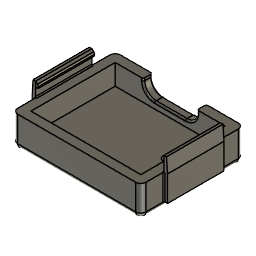
ด้านบน (Autodesk Fusion 360 design; units mm, degrees)
Autodesk Fusion 360 part; units mm, degrees
note: some values were not read from the file. Set by a fixed rule: which sketch regions a step uses.
sketch "Sketch1" plane through (0, 0, 0) normal (0, 0, 1) x (1, 0, 0)
  line L0 (0, 0) -> (21.4, 0)
  line L1 (21.4, 0) -> (21.4, 16.4)
  line L2 (21.4, 16.4) -> (0, 16.4)
  line L3 (0, 16.4) -> (0, 0)
  line L4 (-1.8, -1.8) -> (23.2, -1.8)
  line L5 (23.2, -1.8) -> (23.2, 18.2)
  line L6 (23.2, 18.2) -> (-1.8, 18.2)
  line L7 (-1.8, 18.2) -> (-1.8, -1.8)
  dimension "d1" = 21.4
  dimension "d2" = 16.4
  dimension "d3" = 25
  dimension "d4" = 20
  dimension "d5" = 1.8
  dimension "d6" = 1.8
  constraint horizontal L0
  constraint vertical L1
  constraint horizontal L2
  constraint vertical L3
  constraint coincident L0.start L3.end
  constraint horizontal L4
  constraint vertical L5
  constraint horizontal L6
  constraint vertical L7
  measures "d1" distance of L0.start L0.end
  measures "d2" distance of L0.start L2.end
  measures "d3" distance of L4.start L4.end
  measures "d4" distance of L4.start L6.end
  measures "d5" distance of L3 L7
  measures "d6" distance of L2 L6
extrude "Extrude1" add sketch "Sketch1" along normal blind 6 makes body 1
extrude "Extrude2" add sketch "Sketch1" along normal blind 2 contours L0 L1 L2 L3 bodies 1
fillet "Fillet1" radius 1 7 edges at (23.2, 8.2, 0) (10.7, 18.2, 0) (23.2, 18.2, 3) (23.2, -1.8, 3) (10.7, -1.8, 0) (-1.8, 8.2, 0) (-1.8, -1.8, 3) on bodies 1
fillet "Fillet2" radius 1 2 edges at (-1.5071, 17.9071, 0.2929) (-1.8, 18.2, 3.5) on bodies 1
sketch "Sketch3" plane through (23.2, 0, 0) normal (1, 0, 0) x (0, 1, 0)
  line L0 (-0.8, 6) -> (-0.8, 1)
  line L1 (-0.8, 1) -> (17.2, 1)
  line L2 (17.2, 1) -> (17.2, 6)
  line L3 (17.2, 6) -> (-0.8, 6)
  line L4 (2.7, 6) -> (13.7, 6)
  line L5 (13.7, 6) -> (13.7, 1)
  line L6 (13.7, 1) -> (2.7, 1)
  line L7 (2.7, 1) -> (2.7, 6)
  line L8 (2.7, 6) -> (13.7, 1) construction
  line L9 (13.7, 6) -> (2.7, 1) construction
  point P0 (8.2, 3.5)
  dimension "d15" = 11
  dimension "d16" = 5
  constraint horizontal L4
  constraint perpendicular L4 L5
  constraint parallel L4 L6
  constraint parallel L5 L7
  constraint coincident L8 P0
  constraint coincident L9 P0
  measures "d15" distance of L5.end L6.end
  measures "d16" distance of L4.end L5.end
extrude "Extrude3" add sketch "Sketch3" along normal blind 1 separate body contours L1 L3 L4 L5 L6 L7 makes body 2
sketch "Sketch4" plane through (-1.8, 0, 0) normal (-1, 0, 0) x (0, -1, 0)
  line L0 (-17.2, 6) -> (-17.2, 1)
  line L1 (-17.2, 1) -> (0.8, 1)
  line L2 (0.8, 1) -> (0.8, 6)
  line L3 (0.8, 6) -> (-17.2, 6)
  line L4 (-13.7, 6) -> (-2.7, 6)
  line L5 (-2.7, 6) -> (-2.7, 1)
  line L6 (-2.7, 1) -> (-13.7, 1)
  line L7 (-13.7, 1) -> (-13.7, 6)
  line L8 (-13.7, 6) -> (-2.7, 1) construction
  line L9 (-2.7, 6) -> (-13.7, 1) construction
  point P0 (-8.2, 3.5)
  dimension "d19" = 11
  dimension "d20" = 5
  constraint horizontal L4
  constraint perpendicular L4 L5
  constraint parallel L4 L6
  constraint parallel L5 L7
  constraint coincident L8 P0
  constraint coincident L9 P0
  measures "d19" distance of L5.end L6.end
  measures "d20" distance of L4.end L5.end
extrude "Extrude4" add sketch "Sketch4" along normal blind 1 separate body contours L1 L3 L4 L5 L6 L7 makes body 3
extrude "Extrude5" add 2 faces at (-2.4667, 6.3667, 6) (23.8667, 10.0333, 6) along direction (0, 0, 1) blind 2.8 on bodies 2 3 bodies 1 3 2
sketch "Sketch5" plane through (0, 2.7, 0) normal (0, -1, 0) x (1, 0, 0)
  line L0 (-1.8, 1) -> (-1.8, 6)
  line L1 (-1.8, 6) -> (-1.8, 8.8)
  line L2 (-1.8, 8.8) -> (-2.8, 8.8)
  line L3 (-2.8, 8.8) -> (-2.8, 1)
  line L4 (-2.8, 1) -> (-1.8, 1)
  line L5 (-1.8, 8.8) -> (-1.3, 8.8)
  line L6 (-1.3, 8.8) -> (-1.3, 7.8)
  line L7 (-1.3, 7.8) -> (-1.8, 7.8)
  line L8 (-1.8, 7.8) -> (-1.8, 8.8)
  dimension "d25" = 0.5
  dimension "d26" = 1
  constraint horizontal L5
  constraint vertical L6
  constraint horizontal L7
  constraint vertical L8
  constraint coincident L1.end L2.start
  measures "d25" distance of L1.end L5.end
  measures "d26" distance of L1.end L7.end
sketch "Sketch6" plane through (0, 2.7, 0) normal (0, -1, 0) x (1, 0, 0)
  line L0 (23.2, 6) -> (23.2, 1)
  line L1 (23.2, 1) -> (24.2, 1)
  line L2 (24.2, 1) -> (24.2, 8.8)
  line L3 (24.2, 8.8) -> (23.2, 8.8)
  line L4 (23.2, 8.8) -> (23.2, 6)
  line L5 (23.2, 8.8) -> (22.7, 8.8)
  line L6 (22.7, 8.8) -> (22.7, 7.8)
  line L7 (22.7, 7.8) -> (23.2, 7.8)
  line L8 (23.2, 7.8) -> (23.2, 8.8)
  dimension "d27" = 0.5
  dimension "d28" = 1
  constraint horizontal L5
  constraint vertical L6
  constraint horizontal L7
  constraint vertical L8
  constraint coincident L3.end L4.start
  measures "d27" distance of L3.end L5.end
  measures "d28" distance of L3.end L7.end
extrude "Extrude6" add sketch "Sketch6" sketch "Sketch5" against normal blind 11 separate body contours L4 L5 L6 L7 L8 of sketch 2 contours L1 L5 L6 L7 L8 makes body 4 at (22.7, 6.3667, 8.4667) makes body 5 at (-1.3, 6.3667, 8.4667)
sketch "Sketch7" plane through (0, 2.7, 0) normal (0, -1, 0) x (1, 0, 0)
  line L0 (-1.8, 1) -> (-1.8, 6)
  line L1 (-1.8, 6) -> (-1.8, 8.8)
  line L2 (-1.8, 8.8) -> (-2.8, 8.8)
  line L3 (-2.8, 8.8) -> (-2.8, 1)
  line L4 (-2.8, 1) -> (-1.8, 1)
  line L5 (-1.8, 6) -> (-2.4875, 6)
  line L6 (-2.4875, 6) -> (-2.8, 6)
  line L7 (-2.4875, 5.8364) -> (-2.4875, 1)
  line L8 (-2.4875, 6) -> (-2.3, 8.8)
  line L9 (-2.4875, 5.8364) -> (-2.4875, 6)
  constraint midpoint L2 L8.end
  constraint coincident L0.end L1.start
  constraint perpendicular L0 L5
  constraint coincident L3 L6.end
  constraint perpendicular L3 L6
  constraint coincident L4 L7.end
  constraint perpendicular L4 L7
  constraint perpendicular L5 L9
chamfer "Chamfer1" distance 0.5 angle 45 1 edges at (22.7, 8.2, 8.8) on bodies 4
chamfer "Chamfer2" distance 0.5 angle 45 1 edges at (-1.3, 8.2, 8.8) on bodies 5
fillet "Fillet6" radius 0.5 1 edges at (22.7, 8.2, 8.3) on bodies 4 5
fillet "Fillet6" radius 0.5 1 edges at (-1.3, 8.2, 8.3) on bodies 4 5
extrude "Extrude7" cut sketch "Sketch7" against normal blind 18.339 contours L2 L3 L6 L8 bodies 1
sketch "Sketch8" plane through (0, 2.7, 0) normal (0, -1, 0) x (1, 0, 0)
  line L0 (23.2, 6) -> (23.2, 1)
  line L1 (23.2, 1) -> (24.2, 1)
  line L2 (24.2, 1) -> (24.2, 8.8)
  line L3 (24.2, 8.8) -> (23.2, 8.8)
  line L4 (23.2, 8.8) -> (23.2, 6)
  line L5 (23.8875, 6) -> (23.7, 8.8)
  line L6 (23.2, 6) -> (23.8875, 6)
  line L7 (23.8875, 6) -> (23.8875, 1)
  constraint midpoint L3 L5.end
  constraint coincident L0.start L4.end
  constraint perpendicular L0 L6
  constraint coincident L1 L7.end
  constraint perpendicular L1 L7
extrude "Extrude8" cut sketch "Sketch7" against normal blind 13.909 contours L3 L4 L6 L7 L9 bodies 1
extrude "Extrude9" cut sketch "Sketch8" against normal blind 13.108 contours L1 L2 L3 L5 L7 bodies 1
sketch "Sketch9" plane through (0, 0, 6) normal (0, 0, 1) x (-1, 0, 0)
  line L0 (-23.2, -2.7) -> (-23.2, -13.7)
  line L1 (-23.2, -13.7) -> (-23.2, -17.2)
  arc A0 (-23.2, -17.2) -> (-22.2, -18.2) centre (-22.2, -17.2) ccw
  line L2 (-22.2, -18.2) -> (0.8, -18.2)
  arc A1 (0.8, -18.2) -> (1.8, -17.2) centre (0.8, -17.2) ccw
  line L3 (1.8, -17.2) -> (1.8, -13.7)
  line L4 (1.8, -13.7) -> (1.8, -2.7)
  line L5 (1.8, -2.7) -> (1.8, 0.8)
  arc A2 (1.8, 0.8) -> (0.8, 1.8) centre (0.8, 0.8) ccw
  line L6 (0.8, 1.8) -> (-22.2, 1.8)
  arc A3 (-22.2, 1.8) -> (-23.2, 0.8) centre (-22.2, 0.8) ccw
  line L7 (-23.2, 0.8) -> (-23.2, -2.7)
  line L8 (0, 0) -> (0, -16.4)
  line L9 (0, -16.4) -> (-21.4, -16.4)
  line L10 (-21.4, -16.4) -> (-21.4, 0)
  line L11 (-21.4, 0) -> (0, 0)
  line L12 (-10.7, -16.4) -> (-10.7, -17.3) construction
  line L13 (-15.7, -16.4) -> (-5.7, -16.4)
  line L14 (-5.7, -16.4) -> (-5.7, -18.2)
  line L15 (-5.7, -18.2) -> (-15.7, -18.2)
  line L16 (-15.7, -18.2) -> (-15.7, -16.4)
  line L17 (-15.7, -16.4) -> (-5.7, -18.2) construction
  line L18 (-5.7, -16.4) -> (-15.7, -18.2) construction
  point P0 (-10.7, -17.3)
  dimension "d51" = 0.9
  dimension "d52" = 10
  constraint midpoint L9 L12.start
  constraint perpendicular L9 L12
  constraint horizontal L13
  constraint perpendicular L13 L14
  constraint parallel L13 L15
  constraint parallel L14 L16
  constraint coincident L17 P0
  constraint coincident L18 P0
  constraint coincident P0 L12.end
  measures "d51" distance of L12.start P0
  measures "d52" distance of L14.end L15.end
extrude "Extrude10" cut sketch "Sketch9" against normal blind 2.75 contours L2 L9 L13 L14 L15 L16 bodies 1
sketch "Sketch10" plane through (0, 18.2, 0) normal (0, 1, 0) x (-1, 0, 0)
  line L0 (-15.7, 3.25) -> (-15.7, 6)
  line L1 (-15.7, 6) -> (-22.2, 6)
  line L2 (-22.2, 6) -> (-22.2, 1)
  line L3 (-22.2, 1) -> (0.8, 1)
  line L4 (0.8, 1) -> (0.8, 6)
  line L5 (0.8, 6) -> (-5.7, 6)
  line L6 (-5.7, 6) -> (-5.7, 3.25)
  line L7 (-5.7, 3.25) -> (-15.7, 3.25)
  line L8 (-7.7, 6) -> (-7.7, 5.5) construction
  line L9 (-13.7, 3.25) -> (-7.7, 3.25)
  line L10 (-15.95, 5.5) -> (-5.45, 5.5)
  arc A0 (-15.95, 5.5) -> (-13.7, 3.25) centre (-13.7, 5.5) ccw
  arc A1 (-7.7, 3.25) -> (-5.45, 5.5) centre (-7.7, 5.5) ccw
  line L11 (-15.95, 5.5) -> (-15.95, 6)
  line L12 (-5.45, 5.5) -> (-5.45, 6)
  dimension "d58" = 0.5
  dimension "d71" = 4.5
  dimension "d72" = 4.5
  constraint tangent L9 A1
  constraint tangent L9 A0
  constraint perpendicular L6 L10
  constraint coincident L1 L11.end
  constraint tangent A0 L11
  constraint perpendicular L1 L11
  constraint coincident L5 L12.end
  constraint tangent A1 L12
  constraint perpendicular L5 L12
  measures "d58" distance of L8.start L8.end
  measures "d71" diameter of A0
  measures "d72" diameter of A1
extrude "Extrude11" add sketch "Sketch10" against normal blind 1.8 contours L0 L7 A0 | L6 L7 A1 bodies 1
fillet "Fillet8" radius 0.2 4 edges at (23.2, 13.7, 3.5) (23.2, 2.7, 3.5) (-1.8, 2.7, 3.5) (-1.8, 13.7, 3.5) on bodies 1
fillet "Fillet9" radius 0.2 2 edges at (23.2, 8.2, 6) (-1.8, 8.2, 6) on bodies 1
extrude "Extrude12" cut sketch "Sketch10" against normal blind 1.8 contours L0 L10 A0 | L0 L1 L10 L11 | L6 L10 A1 | L5 L6 L10 L12 bodies 1
fillet "Fillet10" radius 0.3 10 edges at (10.7, 18.2, 3.25) (6.109, 18.2, 3.909) (5.45, 18.2, 5.75) (6.109, 16.4, 3.909) (5.45, 16.4, 5.75) (10.7, 16.4, 3.25) (15.291, 18.2, 3.909) (15.95, 18.2, 5.75) (15.95, 16.4, 5.75) (15.291, 16.4, 3.909) on bodies 1
equation "d3 = 21.4 mm + ( 1.8 * 2 ) * 1 mm"
equation "d4 = 16.4 mm + ( 1.8 * 2 ) * 1 mm"
equation "d15 = 18 mm - ( 3.5 * 2 ) * 1 mm"
equation "d19 = 18 mm - ( 3.5 * 2 ) * 1 mm"
